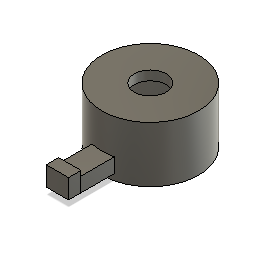
Shell v1 (Autodesk Fusion 360 design; units mm, degrees)
Autodesk Fusion 360 part; units mm, degrees
sketch "Esboço1" plane through (0, 0, 0) normal (0, 1, 0) x (1, 0, 0)
  circle A0 centre (0, 0) radius 16.7
  circle A1 centre (0, 0) radius 14.5
  circle A2 centre (0, 0) radius 5.5
  dimension "d1" = 33.4
  dimension "d2" = 29
  dimension "d12" = 11
  constraint coincident A0.centre A1.centre
  constraint concentric A0 A2
  measures "d1" diameter of A0
  measures "d2" diameter of A1
  measures "d12" diameter of A2
extrude "Extrusão1" add sketch "Esboço1" along normal blind 19.25 contours A0 | A1 | A2 makes body 1
extrude "Extrusão2" cut sketch "Esboço1" along normal blind 16 contours A1 | A2 bodies 1
sketch "Esboço2" plane through (0, 0, 0) normal (0, 0, 1) x (1, 0, 0)
  line L0 (0, 0) -> (-4.5, 0)
  line L1 (-3.85, 7.2) -> (3.85, 7.2)
  line L2 (3.85, 7.2) -> (3.85, 2.2)
  line L3 (3.85, 2.2) -> (-3.85, 2.2)
  line L4 (-3.85, 2.2) -> (-3.85, 7.2)
  line L5 (-3.85, 2.2) -> (3.85, 2.2)
  line L6 (3.85, 2.2) -> (3.85, 8.9)
  line L7 (3.85, 8.9) -> (-3.85, 8.9)
  line L8 (-3.85, 8.9) -> (-3.85, 2.2)
  dimension "d15" = 7.7
  dimension "d16" = 5
  dimension "d17" = 3.85
  dimension "d18" = 2.2
  dimension "d19" = 7.7
  dimension "d20" = 6.7
  constraint coincident L0.start origin
  constraint horizontal L0
  constraint horizontal L1
  constraint vertical L2
  constraint horizontal L3
  constraint vertical L4
  constraint horizontal L5
  constraint vertical L6
  constraint horizontal L7
  constraint vertical L8
  measures "d15" distance of L1.start L1.end
  measures "d16" distance of L1.start L3.end
  measures "d17" distance of L0.start L2
  measures "d18" distance of L0 L3
  measures "d19" distance of L4 L6
  measures "d20" distance of L5 L7
extrude "Extrusão4" cut sketch "Esboço1" along normal blind 22 contours A2 bodies 1
extrude "Extrusão6" add sketch "Esboço2" along normal blind 27.8 contours L1 L2 L3 L4 L5 L6 L8 bodies 1
extrude "Extrusão5" add sketch "Esboço2" along normal blind 4.3 from surface at 27.8 separate body makes body 2
extrude "Extrusão7" cut sketch "Esboço2" along normal up to surface end surface at (14.482, 10.6667, 0.7228) on bodies 1 bodies 1
